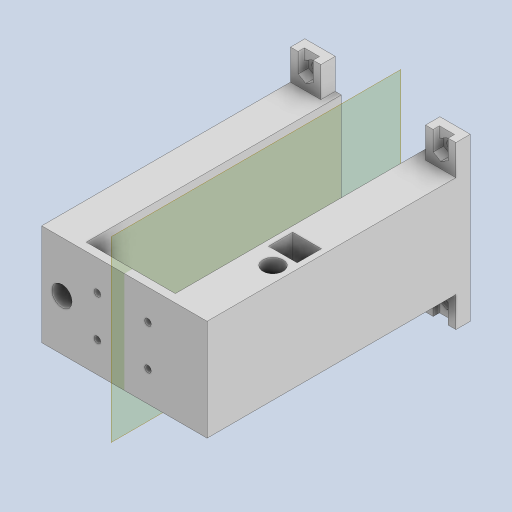
# Autodesk Inventor part: ProbeHead-BaseBody V3
Saved by Autodesk Inventor 2023.2 (Build 272271000, 271)
## iProperties
Created: 2023-12-14
Part Number: ProbeHead-BaseBody V3
Material: Generisch
Document SubType Name: Modeling
Designer: Nils Bade
Density: 1 g/cm^3
Appearance: Vorgabe
Author: Nils Bade
Autodesk Inventor part; units mm, degrees
sketch "S-ProbeHead-BaseSkizze" plane through (0, 0, 0) normal (0, 0, 1) x (1, 0, 0)
  line L0 (-40, 40) -> (40, 40)
  line L1 (40, 40) -> (40, -40)
  line L2 (40, -40) -> (-40, -40)
  line L3 (-40, -40) -> (-40, 40)
  line L4 (-40, 40) -> (40, -40) construction
  line L5 (40, 40) -> (-40, -40) construction
  line L6 (-56.34, 0) -> (58.04, 0) construction
  circle A0 centre (-30, 0) radius 5
  line L7 (0, 83.0683) -> (0, -88.0384) construction
  line L8 (-7.5, 58.6245) -> (-7.5, -60.8735) construction
  line L9 (-16, 21) -> (16, 21) construction
  line L10 (16, 21) -> (16, -21) construction
  line L11 (16, -21) -> (-16, -21) construction
  line L12 (-16, -21) -> (-16, 21) construction
  line L13 (-16, 21) -> (16, -21) construction
  line L14 (16, 21) -> (-16, -21) construction
  circle A1 centre (-12.5, -10) radius 1.65
  circle A2 centre (-12.5, 10) radius 1.65
  circle A3 centre (12.5, -10) radius 1.65
  circle A4 centre (12.5, 10) radius 1.65
  line L15 (-20, 57.6709) -> (-20, -63.5946)
  line L16 (7.5, 58.6245) -> (7.5, -60.8735) construction
  line L17 (20, 57.6709) -> (20, -63.5946)
  line L18 (41.7, 25) -> (-40, 25)
  line L19 (-40, 25) -> (-40, -25)
  line L20 (-40, -25) -> (41.7, -25)
  line L21 (41.7, -25) -> (41.7, 25)
  line L22 (22, 25) -> (22, -25)
  line L23 (-22, -25) -> (-22, 25)
  point P0 (0, 0)
  point P1 (41.7, 0)
  dimension "d1" = 80
  dimension "d2" = 80
  dimension "d4" = 10
  dimension "d6" = 30
  dimension "d20" = 7.5
  dimension "d21" = 32
  dimension "d22" = 42
  dimension "d23" = 3.3
  dimension "d24" = 10
  dimension "d25" = 12.5
  dimension "d26" = 20
  dimension "d27" = 50
  dimension "d30" = 20
  dimension "d31" = 21.7
  dimension "d32" = 2
  dimension "d37" = 2
  constraints: 44 end point, 7 symmetric about line, 6 parallel, 6 point on line, 5 centre point, 5 midpoint, 5 perpendicular, 3 horizontal, 2 vertical, 3 other
  measures "d1" distance of L1.end L2.end
  measures "d2" distance of L0.end L1.end
  measures "d4" diameter of A0
  measures "d6" distance from line of L7 A0.centre
  measures "d20" distance between parallel lines of L7 L8
  measures "d21" distance of L10.end L11.end
  measures "d22" distance of L9.end L10.end
  measures "d23" diameter of A1
  measures "d24" distance from line of L6 A1.centre
  measures "d25" distance from line of L7 A1.centre
  measures "d26" distance between parallel lines of L7 L15
  measures "d27" distance between parallel lines of L20 L18
  measures "d30" distance between parallel lines of L19 L15
  measures "d31" distance between parallel lines of L17 L21
  measures "d32" distance between parallel lines of L17 L22
  measures "d37" distance between parallel lines of L15 L23
extrude "BasePlate" add sketch "S-ProbeHead-BaseSkizze" along normal blind 4 contours L18 L23 L20 L3 | L18 L17 L20 L15 | L15 L20 L23 L18 | L18 L22 L20 L17 | L18 L21 L20 L1 | L1 L20 L22 L18
ref_plane "Endfläche-ProbeHeadarme" through (0, 0, -126) normal (0, 0, 1) x (1, 0, 0)
ref_plane "ProfilDownside" through (0, 0, -56) normal (0, 0, 1) x (1, 0, 0)
extrude "Arms" add sketch "S-ProbeHead-BaseSkizze" against normal up to surface (126 mm away) contours L18 L23 L20 L3 | L18 L21 L20 L1 | L1 L20 L22 L18
ref_plane "Z-UpperBelt" through (0, 0, -36.1) normal (0, 0, 1) x (1, 0, 0)
ref_plane "Z-LowerBelt" through (0, 0, -49.1) normal (0, 0, 1) x (1, 0, 0)
ref_plane "X-Belts" through (26.75, 0, 0) normal (1, 0, 0) x (0, 1, 0)
sketch "S-Tensioners" plane through (-40, -25, 4) normal (0, -1, 0) x (1, 0, 0)
  line L0 (64.75, -47.25) -> (78.95, -47.25)
  line L1 (78.95, -47.25) -> (78.95, -58.95)
  line L2 (78.95, -58.95) -> (64.75, -58.95)
  line L3 (64.75, -58.95) -> (64.75, -47.25)
  line L4 (64.75, -47.25) -> (78.95, -58.95) construction
  line L5 (78.95, -47.25) -> (64.75, -58.95) construction
  line L6 (71.85, -74) -> (71.85, 12.5724) construction
  line L7 (-16.34, -40.1) -> (98.04, -40.1) construction
  line L8 (-16.34, -53.1) -> (98.04, -53.1) construction
  circle A0 centre (74.15, -53.1) radius 2.9
  line L9 (64.75, -34.25) -> (78.95, -34.25)
  line L10 (78.95, -34.25) -> (78.95, -45.95)
  line L11 (78.95, -45.95) -> (64.75, -45.95)
  line L12 (64.75, -45.95) -> (64.75, -34.25)
  line L13 (64.75, -34.25) -> (78.95, -45.95) construction
  line L14 (78.95, -34.25) -> (64.75, -45.95) construction
  circle A1 centre (74.15, -40.1) radius 2.9
  circle A2 centre (74.15, -40.1) radius 5
  circle A3 centre (74.15, -53.1) radius 5
  line L15 (66.75, 41.0869) -> (66.75, -158.5145) construction
  line L16 (78.95, -34.25) -> (64.75, -34.25)
  line L17 (64.75, -34.25) -> (64.75, -33.95)
  line L18 (64.75, -33.95) -> (78.95, -33.95)
  line L19 (78.95, -33.95) -> (78.95, -34.25)
  line L20 (78.95, -58.95) -> (64.75, -58.95)
  line L21 (64.75, -58.95) -> (64.75, -59.25)
  line L22 (64.75, -59.25) -> (78.95, -59.25)
  line L23 (78.95, -59.25) -> (78.95, -58.95)
  point P0 (40, -4)
  point P1 (78.95, -40.1)
  point P2 (78.95, -53.1)
  dimension "d38" = 14.2
  dimension "d39" = 11.7
  dimension "d42" = 5.8
  dimension "d43" = 14.2
  dimension "d44" = 11.7
  dimension "d45" = 5.8
  dimension "d53" = 4.8
  dimension "d54" = 4.8
  dimension "d55" = 10
  dimension "d56" = 10
  dimension "d58" = 7.4
  dimension "d59" = 7.4
  dimension "d79" = 0.3
  dimension "d80" = 0.3
  constraints: 42 end point, 8 parallel, 5 point on line, 4 centre point, 4 coincident, 4 horizontal, 4 perpendicular, 2 midpoint, 1 vertical
  measures "d38" distance of L1.end L2.end
  measures "d39" distance of L0.end L1.end
  measures "d42" diameter of A0
  measures "d43" distance of L10.end L11.end
  measures "d44" distance of L9.end L10.end
  measures "d45" diameter of A1
  measures "d53" distance from line of L10 A1.centre
  measures "d54" distance from line of L1 A0.centre
  measures "d55" diameter of A2
  measures "d56" diameter of A3
  measures "d58" distance from line of L15 A1.centre
  measures "d59" distance from line of L15 A0.centre
  measures "d79" distance between parallel lines of L2 L22
  measures "d80" distance between parallel lines of L16 L18
extrude "Ex-Tensioners1-Holes" cut sketch "S-Tensioners" against normal blind 50 contours A0 | A1
extrude "Ex-Tensioners2-SlideVolume" cut sketch "S-Tensioners" along normal blind 35 from surface at -50 contours L0 L1 A3 L2 L3 | L2 L23 L22 L21 | L1 A3 picked at (78.3167, -53.1)
extrude "Ex-Tensioners3-SlideVolume" cut sketch "S-Tensioners" against normal blind 35 contours L17 L18 L19 L9 | L9 L10 A2 L11 L12 | L10 A2 picked at (78.3167, -40.1)
extrude "Ex-Tensioners4-SrewHead" cut sketch "S-Tensioners" against normal blind 7 contours A3 L1 | L1 A3
extrude "Ex-Tensioners5-SrewHead" cut sketch "S-Tensioners" along normal blind 7 from surface at -50 contours A2 L10 | L10 A2
sketch "S-Anschraubpunkte-ProbeAntenna" plane through (0, 0, -126) normal (0, 0, 1) x (1, 0, 0)
  line L0 (-56.34, 0) -> (58.04, 0) construction
  line L1 (0, 74.3335) -> (0, -68.3114) construction
  line L2 (41.7, 25) -> (-40, 25) projected
  line L3 (41.7, -25) -> (41.7, 25) projected
  line L4 (-40, -25) -> (41.7, -25) projected
  line L5 (-40, 25) -> (-40, -25) projected
  line L6 (41.7, 25) -> (26.7, 25)
  line L7 (26.7, 25) -> (26.7, 40)
  line L8 (26.7, 40) -> (41.7, 40)
  line L9 (41.7, 40) -> (41.7, 25)
  line L10 (22, -25) -> (22, 25) projected
  line L11 (22, 25) -> (22, -25) projected
  line L12 (-22, 25) -> (-22, -25) projected
  line L13 (-22, -25) -> (-22, 25) projected
  line L14 (41.7, 32.5) -> (26.7, 32.5) construction
  line L15 (34.2, 40) -> (34.2, 25) construction
  circle A0 centre (34.2, 32.5) radius 2.15
  circle A1 centre (34.2, 32.5) radius 4 construction
  line L16 (0.85, 53.9557) -> (0.85, -47.9335) construction
  line L17 (-40, 25) -> (-25, 25)
  line L18 (-25, 25) -> (-25, 40)
  line L19 (-25, 40) -> (-40, 40)
  line L20 (-40, 40) -> (-40, 25)
  circle A2 centre (-32.5, 32.5) radius 2.15
  circle A3 centre (-32.5, 32.5) radius 4 construction
  line L21 (41.7, -25) -> (26.7, -25)
  line L22 (26.7, -25) -> (26.7, -40)
  line L23 (26.7, -40) -> (41.7, -40)
  line L24 (41.7, -40) -> (41.7, -25)
  circle A4 centre (34.2, -32.5) radius 2.15
  circle A5 centre (34.2, -32.5) radius 4 construction
  line L25 (-40, -40) -> (-40, -25)
  line L26 (-25, -40) -> (-40, -40)
  line L27 (-40, -25) -> (-25, -25)
  line L28 (-25, -25) -> (-25, -40)
  circle A6 centre (-32.5, -32.5) radius 4 construction
  circle A7 centre (-32.5, -32.5) radius 2.15
  line L29 (34.2, 28.1987) -> (30.475, 30.3494)
  line L30 (30.475, 30.3494) -> (30.475, 40)
  line L31 (30.475, 34.6506) -> (34.2, 36.8013)
  line L32 (34.2, 36.8013) -> (37.925, 34.6506)
  line L33 (37.925, 40) -> (37.925, 30.3494)
  line L34 (37.925, 30.3494) -> (34.2, 28.1987)
  line L35 (34.2, -28.1987) -> (30.475, -30.3494)
  line L36 (30.475, -30.3494) -> (30.475, -40)
  line L37 (30.475, -34.6506) -> (34.2, -36.8013)
  line L38 (34.2, -36.8013) -> (37.925, -34.6506)
  line L39 (37.925, -40) -> (37.925, -30.3494)
  line L40 (37.925, -30.3494) -> (34.2, -28.1987)
  line L41 (-32.5, 28.1987) -> (-28.775, 30.3494)
  line L42 (-28.775, 30.3494) -> (-28.775, 40)
  line L43 (-28.775, 34.6506) -> (-32.5, 36.8013)
  line L44 (-32.5, 36.8013) -> (-36.225, 34.6506)
  line L45 (-36.225, 40) -> (-36.225, 30.3494)
  line L46 (-36.225, 30.3494) -> (-32.5, 28.1987)
  line L47 (-36.225, -40) -> (-36.225, -30.3494)
  line L48 (-32.5, -36.8013) -> (-36.225, -34.6506)
  line L49 (-28.775, -34.6506) -> (-32.5, -36.8013)
  line L50 (-28.775, -30.3494) -> (-28.775, -40)
  line L51 (-32.5, -28.1987) -> (-28.775, -30.3494)
  line L52 (-36.225, -30.3494) -> (-32.5, -28.1987)
  point P0 (0, 0)
  dimension "d46" = 50
  dimension "d67" = 15
  dimension "d68" = 15
  dimension "d69" = 4.3
  dimension "d70" = 8
  dimension "d71" = 81.7
  dimension "d72" = 40.85
  dimension "d75" = 65
  dimension "d76" = 66.7
  dimension "d81" = 7.45
  constraints: 86 end point, 39 symmetric about line, 10 point on line, 8 centre point, 5 coincident, 5 midpoint, 2 parallel, 2 vertical, 1 horizontal, 1 perpendicular, 19 other
  measures "d67" distance of L8.end L2.start
  measures "d68" distance of L7.end L8.end
  measures "d69" diameter of A0
  measures "d70" diameter of A1
  measures "d71" distance between parallel lines of L5 L3
  measures "d72" distance between parallel lines of L3 L16
  measures "d75" distance of A4.centre A0.centre
  measures "d76" distance of A2.centre A0.centre
  measures "d81" distance between parallel lines of L31 L34
extrude "Ex-Anschraubpunkte-Eb1" add sketch "S-Anschraubpunkte-ProbeAntenna" along normal blind 2 contours L2 L7 L8 L30 L29 L34 L33 L9 | L24 L23 L39 L40 L35 L36 L22 L4 | L33 L32 L31 L30 L8 | L23 L36 L37 L38 L39 | L33 L34 L29 L30 L31 L32 | L2 L20 L19 L45 L46 L41 L42 L18 | L38 L37 L36 L35 L40 L39 | L28 L26 L50 L51 L52 L47 L25 L4 | L42 L43 L44 L45 L19 | L42 L41 L46 L45 L44 L43 | L26 L47 L48 L49 L50 | L49 L48 L47 L52 L51 L50
extrude "Ex-Anschraubpunkte-Eb2" add sketch "S-Anschraubpunkte-ProbeAntenna" along normal blind 2 from surface at 2 contours L2 L7 L8 L30 L29 L34 L33 L9 | L24 L23 L39 L40 L35 L36 L22 L4 | L33 L32 L31 L30 L8 | L23 L36 L37 L38 L39 | L2 L20 L19 L45 L46 L41 L42 L18 | L28 L26 L50 L51 L52 L47 L25 L4 | L42 L43 L44 L45 L19 | L26 L47 L48 L49 L50
extrude "Ex-Anschraubpunkte-Eb3" add sketch "S-Anschraubpunkte-ProbeAntenna" along normal blind 3.1 from surface at 4 contours L2 L7 L8 L30 L29 L34 L33 L9 | L24 L23 L39 L40 L35 L36 L22 L4 | L2 L20 L19 L45 L46 L41 L42 L18 | L28 L26 L50 L51 L52 L47 L25 L4
extrude "Ex-Anschraubpunkte-Eb4" [suppressed]
ref_plane "Anschraubpunkt-Spiegelebene" through (0.85, 53.9557, -126) normal (-1, 0, 0) x (0, -1, 0)
ref_plane "ProfilTopSide" through (0, 0, -16) normal (0, 0, 1) x (1, 0, 0)
equation "\"d43\" = d38"
equation "\"d44\" = d39"
equation "\"d45\" = d42"
equation "\"d53\" = d54"
equation "\"d55\" = d56"
equation "\"d58\" = d59"
equation "\"d80\" = d79"
equation "\"d72\" = 0.5 * d71"
